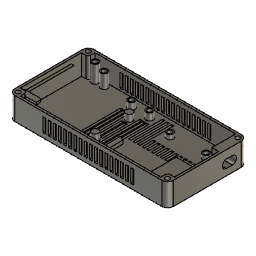
Sensors Case Bottom (Autodesk Fusion 360 design; units mm, degrees)
Autodesk Fusion 360 part; units mm, degrees
note: some values were not read from the file. Set by a fixed rule: which sketch regions a step uses.
(part 1 of 2)
sketch "Sketch1" plane through (0, 0, 0) normal (0, 0, 1) x (1, 0, 0)
  line L0 (65, 35) -> (-65, 35)
  line L1 (-70, 30) -> (-70, -30)
  line L2 (-65, -35) -> (65, -35)
  line L3 (70, -30) -> (70, 30)
  line L4 (70, 35) -> (-70, -35) construction
  line L5 (-70, 35) -> (70, -35) construction
  line L6 (-66, 44.9557) -> (-66, -54.1355) construction
  line L7 (-76.613, 31) -> (75, 31) construction
  line L8 (66, 41.9597) -> (66, -40) construction
  line L9 (75, -31) -> (-75, -31) construction
  line L10 (-62, 35) -> (-65, 35)
  line L11 (-70, 30) -> (-70, 27)
  line L12 (-70, 27) -> (-64, 27)
  line L13 (-62, 29) -> (-62, 35)
  line L14 (-62, 35) -> (-70, 27) construction
  line L15 (-70, 35) -> (-62, 27) construction
  arc A0 (-64, 27) -> (-62, 29) centre (-64, 29) ccw
  arc A1 (-65, 35) -> (-70, 30) centre (-65, 30) ccw
  arc A2 (-65, 35) -> (-70, 30) centre (-65, 30) ccw
  circle A3 centre (-66, 31) radius 3
  arc A4 (70, 30) -> (65, 35) centre (65, 30) ccw
  arc A5 (65, -35) -> (70, -30) centre (65, -30) ccw
  arc A6 (-70, -30) -> (-65, -35) centre (-65, -30) ccw
  line L16 (-64, -27) -> (-70, -27)
  line L17 (-70, -27) -> (-70, -30)
  line L18 (-65, -35) -> (-62, -35)
  line L19 (-62, -35) -> (-62, -29)
  line L20 (-62, -27) -> (-70, -35) construction
  line L21 (-70, -27) -> (-62, -35) construction
  arc A7 (-70, -30) -> (-65, -35) centre (-65, -30) ccw
  arc A8 (-62, -29) -> (-64, -27) centre (-64, -29) ccw
  circle A9 centre (-66, -31) radius 3
  line L22 (0, 0) -> (0, -13) construction
  arc A10 (64, -27) -> (62, -29) centre (64, -29) ccw
  line L23 (70, -27) -> (70, -30)
  line L24 (62, -35) -> (62, -29)
  line L25 (70, 27) -> (64, 27)
  arc A11 (70, 30) -> (65, 35) centre (65, 30) ccw
  line L26 (70, 35) -> (62, 27) construction
  arc A12 (65, -35) -> (70, -30) centre (65, -30) ccw
  line L27 (62, 35) -> (70, 27) construction
  line L28 (70, 30) -> (70, 27)
  arc A13 (65, -35) -> (70, -30) centre (65, -30) ccw
  arc A14 (62, 29) -> (64, 27) centre (64, 29) ccw
  line L29 (65, -35) -> (62, -35)
  line L30 (62, 29) -> (62, 35)
  circle A15 centre (66, -31) radius 3
  arc A16 (70, 30) -> (65, 35) centre (65, 30) ccw
  line L31 (64, -27) -> (70, -27)
  line L32 (62, -27) -> (70, -35) construction
  line L33 (70, 30) -> (70, -30)
  line L34 (62, 35) -> (65, 35)
  circle A17 centre (66, 31) radius 3
  line L35 (70, -27) -> (62, -35) construction
  line L36 (68, 33) -> (-68, 33)
  line L37 (-68, 33) -> (-68, -33)
  line L38 (-68, -33) -> (68, -33)
  line L39 (68, -33) -> (68, 33)
  line L40 (68, 33) -> (-68, -33) construction
  line L41 (-68, 33) -> (68, -33) construction
  point P0 (-66, 31)
  point P1 (-66, -31)
  point P2 (75, -31)
  point P3 (70, 35)
  point P4 (70, -35)
  point P5 (76.613, 31)
  point P6 (66, -31)
  point P7 (66, 44.9557)
  point P8 (66, 31)
  dimension "d1" = 140
  dimension "d2" = 70
  dimension "d3" = 4
  dimension "d4" = 4
  dimension "d5" = 4
  dimension "d6" = 4
  dimension "d7" = 8
  dimension "d8" = 8
  dimension "d9" = 2
  dimension "d10" = 5
  dimension "d11" = 6
  dimension "d12" = 5
  dimension "d13" = 8
  dimension "d14" = 8
  dimension "d15" = 5
  dimension "d16" = 2
  dimension "d17" = 6
  dimension "d20" = 136
  dimension "d21" = 66
  dimension "d211" = 5
  constraint horizontal L0
  constraint perpendicular L0 L1
  constraint parallel L0 L2
  constraint parallel L1 L3
  constraint coincident L4 L22.start
  constraint coincident L5 L22.start
  constraint coincident L22.start origin
  constraint vertical L6
  constraint perpendicular L3 L7
  constraint perpendicular L2 L8
  constraint perpendicular L1 L9
  constraint horizontal L10
  constraint perpendicular L10 L11
  constraint parallel L10 L12
  constraint parallel L11 L13
  constraint coincident L14 P0
  constraint coincident L15 P0
  constraint coincident L7 P0
  constraint coincident L6 P0
  constraint coincident L15.end L13
  constraint coincident L15.end L12
  constraint tangent L13 A0
  constraint tangent L12 A0
  constraint coincident L5.start L10
  constraint coincident L5.start L1
  constraint tangent L10 A1
  constraint tangent L1 A1
  constraint coincident L5.start L0
  constraint coincident L5.start L11
  constraint tangent L0 A2
  constraint tangent L11 A2
  constraint coincident P0 A3.centre
  constraint coincident P3 L0
  constraint coincident P3 L3
  constraint tangent L0 A4
  constraint tangent L3 A4
  constraint coincident L5.end L3
  constraint coincident L5.end L2
  constraint tangent L3 A5
  constraint tangent L2 A5
  constraint equal A4 A5
  constraint coincident L4.end L1
  constraint coincident L4.end L2
  constraint tangent L1 A6
  constraint tangent L2 A6
  constraint equal A4 A6
  constraint horizontal L16
  constraint perpendicular L16 L17
  constraint parallel L16 L18
  constraint parallel L17 L19
  constraint coincident L20 P1
  constraint coincident L21 P1
  constraint coincident L6 P1
  constraint coincident L9 P1
  constraint coincident L4.end L17
  constraint coincident L4.end L18
  constraint tangent L17 A7
  constraint tangent L18 A7
  constraint coincident L20.start L16
  constraint coincident L20.start L19
  constraint tangent L16 A8
  constraint tangent L19 A8
  constraint coincident P1 A9.centre
  constraint vertical L22
  constraint symmetric L5.start L22 P3
  constraint symmetric L4.end L22 P4
  constraint symmetric L6.start L22 P7
  constraint symmetric L7.start L22 P5
  constraint symmetric L9.end L22 P2
  constraint symmetric L10.start L22 L27.start
  constraint symmetric L11.end L22 L25.start
  constraint symmetric L15.end L22 L26.end
  constraint symmetric P0 L22 P8
  constraint symmetric L13.start L22 A14.start
  constraint symmetric L12.end L22 L25.end
  constraint symmetric A0 L22 A14
  constraint symmetric L0.end L22 L0.start
  constraint symmetric L1.start L22 L3.end
  constraint symmetric A1 L22 A16
  constraint symmetric A2 L22 A11
  constraint symmetric A3 L22 A17
  constraint symmetric L1.end L22 L3.start
  constraint symmetric L2.start L22 L2.end
  constraint symmetric A6 L22 A13
  constraint symmetric L20.start L22 L32.start
  constraint symmetric L16.end L22 L23.start
  constraint symmetric L18.end L22 L24.start
  constraint symmetric P1 L22 P6
  constraint symmetric A7 L22 A12
  constraint symmetric L16.start L22 A10.start
  constraint symmetric L19.end L22 A10.end
  constraint symmetric A8 L22 A10
  constraint symmetric A9 L22 A15
  constraint horizontal L36
  constraint perpendicular L36 L37
  constraint parallel L36 L38
  constraint parallel L37 L39
  constraint coincident L40 L22.start
  constraint coincident L41 L22.start
  measures "d1" distance of L4.end L5.end
  measures "d2" distance of L5.start L4.end
  measures "d3" distance of L2 L9
  measures "d4" distance of L1 L6
  measures "d5" distance of L0 L7
  measures "d6" distance of L3 L8
  measures "d7" distance of L11.end L15.end
  measures "d8" distance of L5.start L11.end
  measures "d9" radius of A0
  measures "d10" radius of A2
  measures "d11" diameter of A3
  measures "d12" radius of A4
  measures "d13" distance of L4.end L18.end
  measures "d14" distance of L16.end L4.end
  measures "d15" radius of A7
  measures "d16" radius of A8
  measures "d17" diameter of A9
  measures "d20" distance of L37.end L38.end
  measures "d21" distance of L36.end L37.end
  measures "d211" radius of A1
extrude "Extrude1" add sketch "Sketch1" along normal blind 20 contours L0 L3 A4 L25 A11 L28 L30 A16 L33 L34 A17 L36 L39 | L0 L13 L30 L36 | L0 L1 L10 L11 L12 L13 A1 A2 A3 L36 L37 | L25 A14 L30 A17 L36 L39 | L3 L25 L31 L33 L39 | L12 L13 A0 A3 L36 L37 | L2 L3 A5 L23 L24 A12 A13 L29 A15 L31 L33 L38 L39 | A10 L24 A15 L31 L38 L39 | L1 L12 L16 L37 | L1 L2 A6 L16 L17 L18 L19 A7 A9 L37 L38 | L2 L19 L24 L38 | L16 L19 A8 A9 L37 L38 makes body 1
sketch "Sketch3" plane through (0, 0, 0) normal (0, 0, -1) x (1, 0, 0)
  circle A0 centre (-66, -31) radius 3
  circle A1 centre (66, 31) radius 3
  line L0 (-62, 33) -> (62, 33)
  line L1 (62, 33) -> (62, 29)
  arc A2 (62, 29) -> (64, 27) centre (64, 29) ccw
  line L2 (64, 27) -> (68, 27)
  line L3 (68, 27) -> (68, -27)
  line L4 (68, -27) -> (64, -27)
  arc A3 (64, -27) -> (62, -29) centre (64, -29) ccw
  line L5 (62, -29) -> (62, -33)
  line L6 (62, -33) -> (-62, -33)
  line L7 (-62, -33) -> (-62, -29)
  arc A4 (-62, -29) -> (-64, -27) centre (-64, -29) ccw
  line L8 (-64, -27) -> (-68, -27)
  line L9 (-68, -27) -> (-68, 27)
  line L10 (-68, 27) -> (-64, 27)
  arc A5 (-64, 27) -> (-62, 29) centre (-64, 29) ccw
  line L11 (-62, 29) -> (-62, 33)
  circle A6 centre (66, -31) radius 3
  circle A7 centre (-66, 31) radius 3
  line L12 (-65, -35) -> (65, -35)
  arc A8 (65, -35) -> (70, -30) centre (65, -30) ccw
  line L13 (70, -30) -> (70, 30)
  arc A9 (70, 30) -> (65, 35) centre (65, 30) ccw
  line L14 (65, 35) -> (-65, 35)
  arc A10 (-65, 35) -> (-70, 30) centre (-65, 30) ccw
  line L15 (-70, 30) -> (-70, -30)
  arc A11 (-70, -30) -> (-65, -35) centre (-65, -30) ccw
  line L16 (-68, -35) -> (68, -35)
  line L17 (70, -33) -> (70, 33)
  line L18 (68, 35) -> (-68, 35)
  line L19 (-70, 33) -> (-70, -33)
  line L20 (-70, -35) -> (70, 35) construction
  line L21 (70, -35) -> (-70, 35) construction
  arc A12 (-70, -33) -> (-68, -35) centre (-68, -33) ccw
  arc A13 (-68, 35) -> (-70, 33) centre (-68, 33) ccw
  arc A14 (70, 33) -> (68, 35) centre (68, 33) ccw
  arc A15 (68, -35) -> (70, -33) centre (68, -33) ccw
  dimension "d22" = 140
  dimension "d23" = 70
  dimension "d24" = 2
  constraint horizontal L16
  constraint perpendicular L16 L17
  constraint parallel L16 L18
  constraint parallel L17 L19
  constraint coincident L20 origin
  constraint coincident L21 origin
  constraint coincident L20.start L16
  constraint coincident L20.start L19
  constraint tangent L16 A12
  constraint tangent L19 A12
  constraint coincident L21.end L19
  constraint coincident L21.end L18
  constraint tangent L19 A13
  constraint tangent L18 A13
  constraint equal A12 A13
  constraint coincident L20.end L18
  constraint coincident L20.end L17
  constraint tangent L18 A14
  constraint tangent L17 A14
  constraint equal A12 A14
  constraint coincident L21.start L17
  constraint coincident L21.start L16
  constraint tangent L17 A15
  constraint tangent L16 A15
  constraint equal A12 A15
  measures "d22" distance of L20.end L21.end
  measures "d23" distance of L21.start L20.end
  measures "d24" radius of A12
extrude "Extrude2" add sketch "Sketch3" against normal blind 2 contours L0 L1 A2 L2 L3 L4 A3 L5 L6 L7 A4 L8 L9 L10 A5 L11 | L12 A8 L13 A9 L14 A10 L15 A11 L16 L17 L18 L19 bodies 1
sketch "Sketch22" plane through (0, 0, 2) normal (0, 0, 1) x (-1, 0, 0)
  line L0 (-62, 33) -> (-62, 29)
  arc A0 (-64, 27) -> (-62, 29) centre (-64, 29) ccw
  line L1 (-64, 27) -> (-68, 27)
  line L2 (-68, 27) -> (-68, -27)
  line L3 (-68, -27) -> (-64, -27)
  arc A1 (-62, -29) -> (-64, -27) centre (-64, -29) ccw
  line L4 (-62, -29) -> (-62, -33)
  line L5 (-62, -33) -> (62, -33)
  line L6 (62, -33) -> (62, -29)
  arc A2 (64, -27) -> (62, -29) centre (64, -29) ccw
  line L7 (64, -27) -> (68, -27)
  line L8 (68, -27) -> (68, 27)
  line L9 (68, 27) -> (64, 27)
  arc A3 (62, 29) -> (64, 27) centre (64, 29) ccw
  line L10 (62, 29) -> (62, 33)
  line L11 (62, 33) -> (-62, 33)
  line L12 (-62, 27) -> (-62, 2)
  line L13 (-62, 2) -> (-68, 2)
  line L14 (-68, 2) -> (-68, 27)
  line L15 (-64.3335, 27) -> (-64.3335, 27.5858)
  line L16 (-64.3335, 27.5858) -> (-62.5858, 27.5858)
  line L17 (-62, 27.5858) -> (-62, 27)
  line L18 (-62.5858, 27.5858) -> (-62.5858, 29.0477)
  line L19 (-62.5858, 29.0477) -> (-62, 29.0477)
  line L20 (-62, 29.0477) -> (-62, 27)
  line L21 (-68, 27) -> (-64.3335, 27)
  constraint horizontal L21
  constraint vertical L12
  constraint horizontal L13
  constraint vertical L14
  constraint coincident L1.end L2.start
  constraint vertical L15
  constraint horizontal L16
  constraint vertical L17
  constraint vertical L18
  constraint horizontal L19
  constraint vertical L20
  constraint coincident A0 L16.end
extrude "Extrude21" add sketch "Sketch22" along normal blind 5 contours A0 L1 L2 L12 L13 L14 L17 L20 L21 bodies 1
sketch "Sketch4" plane through (0, 0, 2) normal (0, 0, 1) x (-1, 0, 0)
  line L0 (-62, 33) -> (-62, 2)
  line L1 (-68, 2) -> (-68, -27)
  line L2 (-68, -27) -> (-64, -27)
  arc A0 (-62, -29) -> (-64, -27) centre (-64, -29) ccw
  line L3 (-62, -29) -> (-62, -33)
  line L4 (-62, -33) -> (62, -33)
  line L5 (62, -33) -> (62, -29)
  arc A1 (64, -27) -> (62, -29) centre (64, -29) ccw
  line L6 (64, -27) -> (68, -27)
  line L7 (68, -27) -> (68, 27)
  line L8 (68, 27) -> (64, 27)
  arc A2 (62, 29) -> (64, 27) centre (64, 29) ccw
  line L9 (62, 29) -> (62, 33)
  line L10 (62, 33) -> (-62, 33)
  line L11 (-45, 1.5) -> (-68, 1.5)
  line L12 (-68, 1.5) -> (-68, 0.5)
  line L13 (-68, 0.5) -> (-45, 0.5)
  line L14 (-45, 0.5) -> (-45, 1.5)
  line L15 (-62, 2) -> (-68, 2)
  dimension "d119" = 1
  dimension "d202" = 31.5
  constraint horizontal L11
  constraint vertical L12
  constraint horizontal L13
  constraint vertical L14
  measures "d119" distance of L11.end L12.end
  measures "d202" distance of L10 L11
extrude "Extrude3" add sketch "Sketch4" along normal blind 8.5 contours L1 L11 L12 L13 L14 bodies 1
sketch "Sketch5" plane through (0, 0, 10.5) normal (0, 0, 1) x (-1, 0, 0)
  line L0 (-45, 0.5) -> (-45, 1.5)
  line L1 (-45, 1.5) -> (-68, 1.5)
  line L2 (-68, 1.5) -> (-68, 0.5)
  line L3 (-68, 0.5) -> (-45, 0.5)
  line L4 (-45, 0.5) -> (-68, 0.5)
  line L5 (-68, 0.5) -> (-68, 27)
  line L6 (-68, 27) -> (-64, 27)
  line L7 (-45, 27) -> (-45, 0.5)
  line L8 (-62, 29) -> (-62, 33)
  line L9 (-62, 33) -> (-45, 33)
  line L10 (-45, 33) -> (-45, 27)
  arc A0 (-64, 27) -> (-62, 29) centre (-64, 29) ccw
  point P0 (-68, 27)
  point P1 (-62, 33)
  dimension "d29" = 2
  constraint horizontal L4
  constraint vertical L5
  constraint horizontal L6
  constraint vertical L7
  constraint coincident L0.start L3.end
  constraint vertical L8
  constraint horizontal L9
  constraint vertical L10
  constraint coincident L7.start L6
  constraint tangent L8 A0
  constraint tangent L6 A0
  constraint coincident P0 L5.end
  constraint coincident P1 L8.end
  measures "d29" radius of A0
extrude "Extrude4" add sketch "Sketch5" along normal blind 1 bodies 1
fillet "Fillet1" radius 2 1 edges at (56.5, -0.5, 11.5) on bodies 1
sketch "Sketch26" plane through (0, -35, 0) normal (0, -1, 0) x (1, 0, 0)
  line L0 (65, 0) -> (65, 20)
  line L1 (65, 20) -> (-65, 20)
  line L2 (-65, 20) -> (-65, 0)
  line L3 (-65, 0) -> (65, 0)
  line L4 (0, 0) -> (0, 20) construction
  line L5 (42, 16) -> (-42, 16)
  line L6 (-42, 16) -> (-42, 4)
  line L7 (-42, 4) -> (42, 4)
  line L8 (42, 4) -> (42, 16)
  line L9 (42, 16) -> (-42, 4) construction
  line L10 (-42, 16) -> (42, 4) construction
  line L11 (-40, 16) -> (-40, 4)
  line L12 (-35.4444, 16) -> (-35.4444, 4)
  line L13 (-37.4444, 16) -> (-37.4444, 4)
  line L14 (-30.8889, 16) -> (-30.8889, 4)
  line L15 (-32.8889, 16) -> (-32.8889, 4)
  line L16 (-26.3333, 16) -> (-26.3333, 4)
  line L17 (-28.3333, 16) -> (-28.3333, 4)
  line L18 (-21.7778, 16) -> (-21.7778, 4)
  line L19 (-23.7778, 16) -> (-23.7778, 4)
  line L20 (-17.2222, 16) -> (-17.2222, 4)
  line L21 (-19.2222, 16) -> (-19.2222, 4)
  line L22 (-12.6667, 16) -> (-12.6667, 4)
  line L23 (-14.6667, 16) -> (-14.6667, 4)
  line L24 (-8.1111, 16) -> (-8.1111, 4)
  line L25 (-10.1111, 16) -> (-10.1111, 4)
  line L26 (-3.5556, 16) -> (-3.5556, 4)
  line L27 (-5.5556, 16) -> (-5.5556, 4)
  line L28 (1, 16) -> (1, 4)
  line L29 (-1, 16) -> (-1, 4)
  line L30 (5.5556, 16) -> (5.5556, 4)
  line L31 (3.5556, 16) -> (3.5556, 4)
  line L32 (10.1111, 16) -> (10.1111, 4)
  line L33 (8.1111, 16) -> (8.1111, 4)
  line L34 (14.6667, 16) -> (14.6667, 4)
  line L35 (12.6667, 16) -> (12.6667, 4)
  line L36 (19.2222, 16) -> (19.2222, 4)
  line L37 (17.2222, 16) -> (17.2222, 4)
  line L38 (23.7778, 16) -> (23.7778, 4)
  line L39 (21.7778, 16) -> (21.7778, 4)
  line L40 (28.3333, 16) -> (28.3333, 4)
  line L41 (26.3333, 16) -> (26.3333, 4)
  line L42 (32.8889, 16) -> (32.8889, 4)
  line L43 (30.8889, 16) -> (30.8889, 4)
  line L44 (37.4444, 16) -> (37.4444, 4)
  line L45 (35.4444, 16) -> (35.4444, 4)
  line L46 (42, 16) -> (42, 4)
  line L47 (40, 16) -> (40, 4)
  point P0 (0, 10)
  dimension "d222" = 84
  dimension "d223" = 12
  dimension "d224" = 2
  dimension "d227" = 82
  dimension "d228" = 0
  constraint coincident L4.start origin
  constraint midpoint L1 L4.end
  constraint horizontal L5
  constraint perpendicular L5 L6
  constraint parallel L5 L7
  constraint parallel L6 L8
  constraint coincident L9 P0
  constraint coincident L10 P0
  constraint midpoint L4 P0
  constraint coincident L5 L11.start
  constraint coincident L7 L11.end
  constraint perpendicular L7 L11
  measures "d222" distance of L6.end L7.end
  measures "d223" distance of L5.end L6.end
  measures "d224" distance of L6 L11
extrude "Extrude25" cut sketch "Sketch26" against normal blind 70 contours L5 L7 L44 L47 | L5 L7 L42 L45 | L5 L7 L40 L43 | L5 L7 L38 L41 | L5 L7 L36 L39 | L5 L7 L34 L37 | L5 L7 L32 L35 | L5 L7 L30 L33 | L5 L7 L28 L31 | L5 L7 L26 L29 | L5 L7 L24 L27 | L5 L7 L22 L25 | L5 L7 L20 L23 | L5 L7 L18 L21 | L5 L7 L16 L19 | L5 L7 L14 L17 | L5 L7 L12 L15 | L5 L7 L11 L13 bodies 1
sketch "Sketch9" plane through (0, 0, 2) normal (0, 0, 1) x (-1, 0, 0)
  line L0 (-68, 1.5) -> (-45, 1.5)
  line L1 (-45, 1.5) -> (-45, 0.5)
  line L2 (-45, 0.5) -> (-68, 0.5)
  line L3 (-68, 0.5) -> (-68, -27)
  line L4 (-68, -27) -> (-64, -27)
  arc A0 (-62, -29) -> (-64, -27) centre (-64, -29) ccw
  line L5 (-62, -29) -> (-62, -33)
  line L6 (-62, -33) -> (62, -33)
  line L7 (62, -33) -> (62, -29)
  arc A1 (64, -27) -> (62, -29) centre (64, -29) ccw
  line L8 (64, -27) -> (68, -27)
  line L9 (68, -27) -> (68, 27)
  line L10 (68, 27) -> (64, 27)
  arc A2 (62, 29) -> (64, 27) centre (64, 29) ccw
  line L11 (62, 29) -> (62, 33)
  line L12 (62, 33) -> (-62, 33)
  line L13 (-62, 33) -> (-62, 2)
  line L14 (-68, 2) -> (-68, 1.5)
  circle A3 centre (50, -29) radius 2
  circle A4 centre (50, -29) radius 3
  line L15 (-62, 2) -> (-68, 2)
  dimension "d86" = 4
  dimension "d87" = 6
  dimension "d142" = 4
  dimension "d143" = 12
  constraint concentric A3 A4
  measures "d86" diameter of A3
  measures "d87" diameter of A4
  measures "d142" distance of L6 A3.centre
  measures "d143" distance of L7 A3.centre
extrude "Extrude9" add sketch "Sketch9" along normal blind 12 separate body contours A4 makes body 2
sketch "Sketch10" plane through (-68, 0, 0) normal (1, 0, 0) x (0, 1, 0)
  line L0 (-27, 2) -> (27, 2)
  line L1 (27, 2) -> (27, 20)
  line L2 (27, 20) -> (-27, 20)
  line L3 (-27, 20) -> (-27, 2)
  line L4 (-25, 14) -> (18, 14)
  line L5 (18, 14) -> (18, 16)
  line L6 (18, 16) -> (-25, 16)
  line L7 (-25, 16) -> (-25, 14)
  dimension "d90" = 2
  dimension "d91" = 43
  dimension "d92" = 2
  dimension "d96" = 4
  constraint horizontal L4
  constraint vertical L5
  constraint horizontal L6
  constraint vertical L7
  measures "d90" distance of L3 L6.end
  measures "d91" distance of L5.end L6.end
  measures "d92" distance of L4.start L6.end
  measures "d96" distance of L2 L6
extrude "Extrude10" add sketch "Sketch10" along normal blind 2.5 contours L4 L5 L6 L7 bodies 1
chamfer "Chamfer1" distance 2 angle 45 1 edges at (-65.5, -3.5, 14) on bodies 1
sketch "Sketch11" plane through (0, 0, 2) normal (0, 0, 1) x (-1, 0, 0)
  line L0 (-68, 1.5) -> (-45, 1.5)
  line L1 (-45, 1.5) -> (-45, 0.5)
  line L2 (-45, 0.5) -> (-68, 0.5)
  line L3 (-68, 0.5) -> (-68, -27)
  line L4 (-68, -27) -> (-64, -27)
  arc A0 (-62, -29) -> (-64, -27) centre (-64, -29) ccw
  line L5 (-62, -29) -> (-62, -33)
  line L6 (-62, -33) -> (62, -33)
  line L7 (62, -33) -> (62, -29)
  arc A1 (64, -27) -> (62, -29) centre (64, -29) ccw
  line L8 (64, -27) -> (68, -27)
  line L9 (68, -27) -> (68, 27)
  line L10 (68, 27) -> (64, 27)
  arc A2 (62, 29) -> (64, 27) centre (64, 29) ccw
  line L11 (62, 29) -> (62, 33)
  line L12 (62, 33) -> (-62, 33)
  line L13 (-62, 33) -> (-62, 2)
  line L14 (-68, 2) -> (-68, 1.5)
  circle A3 centre (21.9294, -25) radius 2
  circle A4 centre (5.9294, -25) radius 2
  circle A5 centre (5.9294, -25) radius 3
  circle A6 centre (21.9294, -25) radius 3
  circle A7 centre (5.9294, 25) radius 2
  circle A8 centre (5.9294, 25) radius 3
  circle A9 centre (21.9294, 25) radius 2
  circle A10 centre (21.9294, 25) radius 3
  line L15 (5.9294, 25) -> (5.9294, -25) construction
  line L16 (21.9294, -25) -> (21.9294, 25) construction
  line L17 (0, 0) -> (27, 0) construction
  line L18 (-62, 2) -> (-68, 2)
  point P0 (21.9294, 0)
  point P1 (5.9294, 0)
  dimension "d97" = 4
  dimension "d98" = 4
  dimension "d99" = 6
  dimension "d100" = 6
  dimension "d101" = 4
  dimension "d102" = 6
  dimension "d103" = 4
  dimension "d104" = 6
  dimension "d151" = 16
  dimension "d154" = 25
  dimension "d155" = 25
  constraint concentric A4 A5
  constraint concentric A3 A6
  constraint concentric A7 A8
  constraint concentric A9 A10
  constraint coincident A7.centre A8.centre
  constraint coincident A4.centre A5.centre
  constraint vertical L15
  constraint coincident A3.centre A6.centre
  constraint coincident A9.centre A10.centre
  constraint vertical L16
  constraint coincident L17.start origin
  constraint horizontal L17
  constraint midpoint L16 P0
  constraint midpoint L15 P1
  constraint coincident L17 P0
  constraint coincident L17 P1
  measures "d97" diameter of A3
  measures "d98" diameter of A4
  measures "d99" diameter of A5
  measures "d100" diameter of A6
  measures "d101" diameter of A7
  measures "d102" diameter of A8
  measures "d103" diameter of A9
  measures "d104" diameter of A10
  measures "d151" distance of L15 L16
  measures "d154" distance of A4.centre P1
  measures "d155" distance of A3.centre L17
extrude "Extrude11" add sketch "Sketch11" along normal blind 6 contours A5 | A6 | A8 | A10 bodies 1
sketch "Sketch12" plane through (0, 0, 2) normal (0, 0, 1) x (-1, 0, 0)
  circle A0 centre (21.9294, -25) radius 3
  circle A1 centre (5.9294, -25) radius 3
  line L0 (-68, 1.5) -> (-45, 1.5)
  line L1 (-45, 1.5) -> (-45, 0.5)
  line L2 (-45, 0.5) -> (-68, 0.5)
  line L3 (-68, 0.5) -> (-68, -27)
  line L4 (-68, -27) -> (-64, -27)
  arc A2 (-62, -29) -> (-64, -27) centre (-64, -29) ccw
  line L5 (-62, -29) -> (-62, -33)
  line L6 (-62, -33) -> (62, -33)
  line L7 (62, -33) -> (62, -29)
  arc A3 (64, -27) -> (62, -29) centre (64, -29) ccw
  line L8 (64, -27) -> (68, -27)
  line L9 (68, -27) -> (68, 27)
  line L10 (68, 27) -> (64, 27)
  arc A4 (62, 29) -> (64, 27) centre (64, 29) ccw
  line L11 (62, 29) -> (62, 33)
  line L12 (62, 33) -> (-62, 33)
  line L13 (-62, 33) -> (-62, 2)
  line L14 (-68, 2) -> (-68, 1.5)
  circle A5 centre (5.9294, 25) radius 3
  circle A6 centre (21.9294, 25) radius 3
  circle A7 centre (13.9294, -15) radius 3
  circle A8 centre (13.9294, 15) radius 3
  line L15 (5.9294, 25) -> (21.9294, 25) construction
  line L16 (13.9294, 25) -> (13.9294, 15) construction
  line L17 (5.9294, -25) -> (21.9294, -25) construction
  line L18 (21.9294, -25) -> (13.9294, -25)
  line L19 (13.9294, -15) -> (13.9294, -25) construction
  line L20 (-62, 2) -> (-68, 2)
  dimension "d115" = 6
  dimension "d116" = 6
  dimension "d153" = 10
  dimension "d156" = 10
  constraint coincident A5.centre L15.start
  constraint coincident A6.centre L15.end
  constraint midpoint L15 L16.start
  constraint coincident A8.centre L16.end
  constraint perpendicular L15 L16
  constraint coincident A1.centre L17.start
  constraint coincident A0.centre L17.end
  constraint midpoint L17 L18.end
  constraint coincident A7.centre L19.start
  constraint perpendicular L17 L19
  measures "d115" diameter of A7
  measures "d116" diameter of A8
  measures "d153" distance of A7.centre L17
  measures "d156" distance of A8.centre L15
extrude "Extrude12" add sketch "Sketch12" along normal blind 6 contours A7 | A8 bodies 1
sketch "Sketch13" plane through (0, 0, 20) normal (0, 0, 1) x (-1, 0, 0)
  line L0 (-62, 33) -> (62, 33)
  line L1 (62, 33) -> (62, 29)
  arc A0 (62, 29) -> (64, 27) centre (64, 29) ccw
  line L2 (64, 27) -> (68, 27)
  line L3 (68, 27) -> (68, -27)
  line L4 (68, -27) -> (64, -27)
  arc A1 (64, -27) -> (62, -29) centre (64, -29) ccw
  line L5 (62, -29) -> (62, -33)
  line L6 (62, -33) -> (-62, -33)
  line L7 (-62, -33) -> (-62, -29)
  arc A2 (-62, -29) -> (-64, -27) centre (-64, -29) ccw
  line L8 (-64, -27) -> (-68, -27)
  line L9 (-68, -27) -> (-68, 27)
  line L10 (-68, 27) -> (-64, 27)
  arc A3 (-64, 27) -> (-62, 29) centre (-64, 29) ccw
  line L11 (-62, 29) -> (-62, 33)
  circle A4 centre (-66, -31) radius 3
  circle A5 centre (66, -31) radius 3
  circle A6 centre (-66, 31) radius 3
  circle A7 centre (66, 31) radius 3
  line L12 (-65, -35) -> (65, -35)
  arc A8 (65, -35) -> (70, -30) centre (65, -30) ccw
  line L13 (70, -30) -> (70, 30)
  arc A9 (70, 30) -> (65, 35) centre (65, 30) ccw
  line L14 (65, 35) -> (-65, 35)
  arc A10 (-65, 35) -> (-70, 30) centre (-65, 30) ccw
  line L15 (-70, 30) -> (-70, -30)
  arc A11 (-70, -30) -> (-65, -35) centre (-65, -30) ccw
  circle A12 centre (66, -31) radius 2
  circle A13 centre (66, 31) radius 2
  circle A14 centre (-66, 31) radius 2
  circle A15 centre (-66, -31) radius 2
  dimension "d121" = 4
  dimension "d122" = 4
  dimension "d123" = 4
  dimension "d124" = 4
  constraint concentric A5 A12
  constraint concentric A7 A13
  constraint concentric A6 A14
  constraint concentric A4 A15
  measures "d121" diameter of A12
  measures "d122" diameter of A13
  measures "d123" diameter of A14
  measures "d124" diameter of A15
extrude "Extrude13" add sketch "Sketch13" against normal blind 6 contours A4 | A5 | A6 | A7 bodies 1
chamfer "Chamfer2" distance 1 angle 45 4 edges at (-64.1353, -30.2768, 14) (-64.1353, 31.7232, 14) (67.8647, -30.2768, 14) (67.8647, 31.7232, 14) on bodies 1
sketch "Sketch16" plane through (0, 0, 2) normal (0, 0, 1) x (-1, 0, 0)
  circle A0 centre (13.9294, -15) radius 3
  circle A1 centre (21.9294, -25) radius 3
  circle A2 centre (5.9294, -25) radius 3
  line L0 (-68, 1.5) -> (-45, 1.5)
  line L1 (-45, 1.5) -> (-45, 0.5)
  line L2 (-45, 0.5) -> (-68, 0.5)
  line L3 (-68, 0.5) -> (-68, -27)
  line L4 (-68, -27) -> (-64, -27)
  arc A3 (-62, -29) -> (-64, -27) centre (-64, -29) ccw
  line L5 (-62, -29) -> (-62, -33)
  line L6 (-62, -33) -> (62, -33)
  line L7 (62, -33) -> (62, -29)
  arc A4 (64, -27) -> (62, -29) centre (64, -29) ccw
  line L8 (64, -27) -> (68, -27)
  line L9 (68, -27) -> (68, 27)
  line L10 (68, 27) -> (64, 27)
  arc A5 (62, 29) -> (64, 27) centre (64, 29) ccw
  line L11 (62, 29) -> (62, 33)
  line L12 (62, 33) -> (-62, 33)
  line L13 (-62, 33) -> (-62, 2)
  line L14 (-68, 2) -> (-68, 1.5)
  circle A6 centre (5.9294, 25) radius 3
  circle A7 centre (21.9294, 25) radius 3
  line L15 (33.1094, 24.8906) -> (29.1094, 24.8906)
  line L16 (29.1094, 24.8906) -> (29.1094, 28.8906)
  line L17 (29.1094, 28.8906) -> (33.1094, 28.8906)
  line L18 (33.1094, 28.8906) -> (33.1094, 24.8906)
  line L19 (33.1094, 24.8906) -> (29.1094, 28.8906) construction
  line L20 (29.1094, 24.8906) -> (33.1094, 28.8906) construction
  line L21 (33.1094, 26.8906) -> (32.1094, 26.8906)
  line L22 (31.1094, 25.8906) -> (31.1094, 24.8906)
  arc A8 (32.1094, 26.8906) -> (31.1094, 25.8906) centre (32.1094, 25.8906) ccw
  circle A9 centre (13.9294, 15) radius 3
  line L23 (-62, 2) -> (-68, 2)
  point P0 (31.1094, 26.8906)
  dimension "d134" = 1
  constraint horizontal L15
  constraint perpendicular L15 L16
  constraint parallel L15 L17
  constraint parallel L16 L18
  constraint coincident L19 P0
  constraint coincident L20 P0
  constraint midpoint L18 L21.start
  constraint midpoint L15 L22.end
  constraint tangent L22 A8
  constraint tangent L21 A8
  measures "d134" radius of A8
extrude "Extrude15" add sketch "Sketch16" along normal blind 2 contours L15 L16 L17 L18 L21 L22 A8 bodies 1
chamfer "Chamfer3" distance 2 angle 45 4 edges at (-29.1094, -26.8906, 2) (-30.1094, -24.8906, 2) (-31.1094, -28.8906, 2) (-33.1094, -27.8906, 2) on bodies 1
sketch "Sketch17" plane through (0, 0, 2) normal (0, 0, 1) x (-1, 0, 0)
  circle A0 centre (21.9294, 25) radius 3
  circle A1 centre (5.9294, 25) radius 3
  line L0 (-68, 1.5) -> (-45, 1.5)
  line L1 (-45, 1.5) -> (-45, 0.5)
  line L2 (-45, 0.5) -> (-68, 0.5)
  line L3 (-68, 0.5) -> (-68, -27)
  line L4 (-68, -27) -> (-64, -27)
  arc A2 (-62, -29) -> (-64, -27) centre (-64, -29) ccw
  line L5 (-62, -29) -> (-62, -33)
  line L6 (-62, -33) -> (62, -33)
  line L7 (62, -33) -> (62, -29)
  arc A3 (64, -27) -> (62, -29) centre (64, -29) ccw
  line L8 (64, -27) -> (68, -27)
  line L9 (68, -27) -> (68, 27)
  line L10 (68, 27) -> (64, 27)
  arc A4 (62, 29) -> (64, 27) centre (64, 29) ccw
  line L11 (62, 29) -> (62, 33)
  line L12 (62, 33) -> (-62, 33)
  line L13 (-62, 33) -> (-62, 2)
  line L14 (-68, 2) -> (-68, 1.5)
  circle A5 centre (5.9294, -25) radius 3
  circle A6 centre (21.9294, -25) radius 3
  circle A7 centre (13.9294, -15) radius 3
  line L15 (31.1094, 25.8906) -> (31.1094, 22.8906)
  line L16 (31.1094, 22.8906) -> (27.1094, 22.8906)
  line L17 (27.1094, 22.8906) -> (27.1094, 30.8906)
  line L18 (27.1094, 30.8906) -> (35.1094, 30.8906)
  line L19 (35.1094, 30.8906) -> (35.1094, 26.8906)
  line L20 (35.1094, 26.8906) -> (32.1094, 26.8906)
  arc A8 (32.1094, 26.8906) -> (31.1094, 25.8906) centre (32.1094, 25.8906) ccw
  line L21 (64, 28) -> (53, 28)
  line L22 (53, 28) -> (53, 27)
  line L23 (53, 27) -> (64, 27)
  line L24 (64, 27) -> (64, 28)
  circle A9 centre (13.9294, 15) radius 3
  line L25 (-62, 2) -> (-68, 2)
  constraint horizontal L21
  constraint vertical L22
  constraint horizontal L23
  constraint vertical L24
extrude "Extrude16" add sketch "Sketch17" along normal blind 13 contours A4 L21 L22 L23 bodies 1
sketch "Sketch18" plane through (0, 0, 15) normal (0, 0, 1) x (-1, 0, 0)
  line L0 (62.2679, 28) -> (53, 28)
  line L1 (53, 28) -> (53, 27)
  line L2 (53, 27) -> (64, 27)
  arc A0 (62.2679, 28) -> (64, 27) centre (64, 29) ccw
  line L3 (53, 28) -> (68, 28)
  line L4 (68, 28) -> (68, 23)
  line L5 (68, 23) -> (53, 23)
  line L6 (53, 23) -> (53, 28)
  dimension "d146" = 15
  dimension "d147" = 5
  constraint horizontal L3
  constraint vertical L4
  constraint horizontal L5
  constraint vertical L6
  constraint coincident L0.end L1.start
  measures "d146" distance of L0.end L3.end
  measures "d147" distance of L0.end L5.end
extrude "Extrude17" add sketch "Sketch18" along normal blind 2 bodies 1
chamfer "Chamfer4" distance 2 angle 45 1 edges at (-59.75, -23, 15) on bodies 1
sketch "Sketch19" plane through (0, 0, 2) normal (0, 0, 1) x (-1, 0, 0)
  line L0 (31.1094, 25.8906) -> (31.1094, 22.8906)
  line L1 (31.1094, 22.8906) -> (27.1094, 22.8906)
  line L2 (27.1094, 22.8906) -> (27.1094, 30.8906)
  line L3 (27.1094, 30.8906) -> (35.1094, 30.8906)
  line L4 (35.1094, 30.8906) -> (35.1094, 26.8906)
  line L5 (35.1094, 26.8906) -> (32.1094, 26.8906)
  arc A0 (32.1094, 26.8906) -> (31.1094, 25.8906) centre (32.1094, 25.8906) ccw
  circle A1 centre (13.9294, 15) radius 3
  circle A2 centre (13.9294, -15) radius 3
  circle A3 centre (21.9294, -25) radius 3
  circle A4 centre (5.9294, -25) radius 3
  line L6 (68, 27) -> (53, 27)
  line L7 (53, 27) -> (53, 28)
  line L8 (53, 28) -> (62.2679, 28)
  arc A5 (62, 29) -> (62.2679, 28) centre (64, 29) ccw
  line L9 (62, 29) -> (62, 33)
  line L10 (62, 33) -> (-62, 33)
  line L11 (-62, 33) -> (-62, 2)
  line L12 (-68, 2) -> (-68, 1.5)
  line L13 (-68, 1.5) -> (-45, 1.5)
  line L14 (-45, 1.5) -> (-45, 0.5)
  line L15 (-45, 0.5) -> (-68, 0.5)
  line L16 (-68, 0.5) -> (-68, -27)
  line L17 (-68, -27) -> (-64, -27)
  arc A6 (-62, -29) -> (-64, -27) centre (-64, -29) ccw
  line L18 (-62, -29) -> (-62, -33)
  line L19 (-62, -33) -> (62, -33)
  line L20 (62, -33) -> (62, -29)
  arc A7 (64, -27) -> (62, -29) centre (64, -29) ccw
  line L21 (64, -27) -> (68, -27)
  line L22 (68, -27) -> (68, 27)
  circle A8 centre (5.9294, 25) radius 3
  circle A9 centre (21.9294, 25) radius 3
  circle A10 centre (-49.5, -19.5) radius 2
  circle A11 centre (-49.5, -19.5) radius 3
  circle A12 centre (-17.5, -19.5) radius 2
  circle A13 centre (-17.5, -19.5) radius 3
  line L23 (-62, 2) -> (-68, 2)
  dimension "d165" = 4
  dimension "d166" = 6
  dimension "d167" = 4
  dimension "d168" = 6
  dimension "d169" = 32
  dimension "d170" = 13.5
  dimension "d171" = 12.5
  dimension "d172" = 13.5
  constraint concentric A10 A11
  constraint concentric A12 A13
  measures "d165" diameter of A10
  measures "d166" diameter of A11
  measures "d167" diameter of A12
  measures "d168" diameter of A13
  measures "d169" distance of A10.centre A12.centre
  measures "d170" distance of L19 A10.centre
  measures "d171" distance of L18 A10.centre
  measures "d172" distance of L19 A12.centre
extrude "Extrude18" add sketch "Sketch19" along normal blind 4 contours A11 | A13 bodies 1
sketch "Sketch20" plane through (0, 0, 2) normal (0, 0, 1) x (-1, 0, 0)
  circle A0 centre (-17.5, -19.5) radius 3
  line L0 (31.1094, 25.8906) -> (31.1094, 22.8906)
  line L1 (31.1094, 22.8906) -> (27.1094, 22.8906)
  line L2 (27.1094, 22.8906) -> (27.1094, 30.8906)
  line L3 (27.1094, 30.8906) -> (35.1094, 30.8906)
  line L4 (35.1094, 30.8906) -> (35.1094, 26.8906)
  line L5 (35.1094, 26.8906) -> (32.1094, 26.8906)
  arc A1 (32.1094, 26.8906) -> (31.1094, 25.8906) centre (32.1094, 25.8906) ccw
  circle A2 centre (13.9294, 15) radius 3
  circle A3 centre (13.9294, -15) radius 3
  circle A4 centre (21.9294, -25) radius 3
  circle A5 centre (5.9294, -25) radius 3
  line L6 (68, 27) -> (53, 27)
  line L7 (53, 27) -> (53, 28)
  line L8 (53, 28) -> (62.2679, 28)
  arc A6 (62, 29) -> (62.2679, 28) centre (64, 29) ccw
  line L9 (62, 29) -> (62, 33)
  line L10 (62, 33) -> (-62, 33)
  line L11 (-62, 33) -> (-62, 2)
  line L12 (-68, 2) -> (-68, 1.5)
  line L13 (-68, 1.5) -> (-45, 1.5)
  line L14 (-45, 1.5) -> (-45, 0.5)
  line L15 (-45, 0.5) -> (-68, 0.5)
  line L16 (-68, 0.5) -> (-68, -27)
  line L17 (-68, -27) -> (-64, -27)
  arc A7 (-62, -29) -> (-64, -27) centre (-64, -29) ccw
  line L18 (-62, -29) -> (-62, -33)
  line L19 (-62, -33) -> (62, -33)
  line L20 (62, -33) -> (62, -29)
  arc A8 (64, -27) -> (62, -29) centre (64, -29) ccw
  line L21 (64, -27) -> (68, -27)
  line L22 (68, -27) -> (68, 27)
  circle A9 centre (5.9294, 25) radius 3
  circle A10 centre (21.9294, 25) radius 3
  circle A11 centre (-49.5, -19.5) radius 3
  line L23 (-68, -27) -> (-64, -27)
  line L24 (-64, -27) -> (-64, -12)
  line L25 (-64, -12) -> (-68, -12)
  line L26 (-68, -12) -> (-68, -27)
  line L27 (-64, -12) -> (-62, -12)
  line L28 (-62, -12) -> (-62, -14.5)
  line L29 (-62, -14.5) -> (-64, -14.5)
  line L30 (-64, -14.5) -> (-64, -12)
  line L31 (-62, -24.55) -> (-64, -24.55)
  line L32 (-62, -24.55) -> (-64, -24.55)
  line L33 (-64, -24.55) -> (-64, -29.55)
  line L34 (-64, -29.55) -> (-62, -29.55)
  line L35 (-62, -29.55) -> (-62, -24.55)
  line L36 (-62, -24.55) -> (-64, -24.55)
  line L37 (-64, -24.55) -> (-64, -14.5)
  line L38 (-64, -14.5) -> (-62, -14.5)
  line L39 (-62, -14.5) -> (-62, -24.55)
  line L40 (-62, 2) -> (-68, 2)
  dimension "d181" = 4
  dimension "d182" = 15
  dimension "d185" = 2
  dimension "d186" = 2.5
  dimension "d188" = 2
  dimension "d189" = 5
  constraint horizontal L23
  constraint vertical L24
  constraint horizontal L25
  constraint vertical L26
  constraint coincident L16.end L17.start
  constraint horizontal L27
  constraint vertical L28
  constraint horizontal L29
  constraint vertical L30
  constraint coincident L24 L31.end
  constraint perpendicular L24 L31
  constraint horizontal L32
  constraint vertical L33
  constraint horizontal L34
  constraint vertical L35
  constraint horizontal L36
  constraint vertical L37
  constraint horizontal L38
  constraint vertical L39
  measures "d181" distance of L16.end L17.end
  measures "d182" distance of L16.end L25.end
  measures "d185" distance of L24.end L27.end
  measures "d186" distance of L24.end L29.end
  measures "d188" distance of L31.start L31.end
  measures "d189" distance of L31.start L34.end
extrude "Extrude19" add sketch "Sketch20" along normal blind 18 contours A7 L24 L31 L32 L33 L35 L36 | L16 L17 L23 L24 L25 L26 L30 L33 L37 | L24 L29 L31 L32 L36 L37 L38 L39 | L24 L27 L28 L29 L30 L38 bodies 1
sketch "Sketch7" plane through (70, 0, 0) normal (1, 0, 0) x (0, 1, 0)
  line L0 (30, 0) -> (30, 20)
  line L1 (30, 20) -> (-30, 20)
  line L2 (-30, 20) -> (-30, 0)
  line L3 (-30, 0) -> (30, 0)
  line L4 (19.5, 20) -> (19.5, 0) construction
  line L5 (13.25, 9.25) -> (46, 9.25) construction
  line L6 (16.75, 7.25) -> (22.35, 7.25)
  arc A0 (22.35, 7.25) -> (22.35, 11.25) centre (22.35, 9.25) ccw
  line L7 (22.35, 11.25) -> (16.75, 11.25)
  arc A1 (16.75, 11.25) -> (16.75, 7.25) centre (16.75, 9.25) ccw
  line L8 (16.75, 9.25) -> (22.35, 9.25) construction
  line L9 (16.9, 5.6) -> (22.1, 5.6)
  arc A2 (22.1, 5.6) -> (22.1, 12.9) centre (22.1, 9.25) ccw
  line L10 (22.1, 12.9) -> (16.9, 12.9)
  arc A3 (16.9, 12.9) -> (16.9, 5.6) centre (16.9, 9.25) ccw
  line L11 (16.9, 9.25) -> (22.1, 9.25) construction
  point P0 (19.5, 9.25)
  point P1 (19.5, 9.25)
  dimension "d47" = 9.25
  dimension "d48" = 10.5
  dimension "d49" = 2.85
  dimension "d50" = 2
  dimension "d51" = 5.6
  dimension "d179" = 7.3
  dimension "d180" = 2.6
  constraint coincident L1 L4.start
  constraint perpendicular L1 L4
  constraint coincident L3 L4.end
  constraint perpendicular L4 L5
  constraint tangent L6 A0
  constraint tangent A0 L7
  constraint parallel L6 L7
  constraint tangent L7 A1
  constraint tangent L6 A1
  constraint perpendicular L4 L8
  constraint coincident L5 P1
  constraint coincident L4 P1
  constraint tangent L9 A2
  constraint tangent A2 L10
  constraint parallel L9 L10
  constraint tangent L10 A3
  constraint tangent L9 A3
  constraint coincident L5 A2.centre
  constraint perpendicular L4 L11
  constraint coincident P1 P0
  constraint midpoint L11 P1
  constraint coincident L8 A2.centre
  constraint midpoint L5.start A3
  measures "d47" distance of L3 L5
  measures "d48" distance of L0 L4
  measures "d49" distance of A0.centre P1
  measures "d50" distance of A0.end A0.centre
  measures "d51" distance of A1.centre A0.centre
  measures "d179" diameter of A2
  measures "d180" distance of P1 A2.centre
extrude "Extrude6" cut sketch "Sketch7" against normal blind 8 contours L6 A0 L7 A1 | L9 A2 L10 A3 bodies 1
sketch "Sketch21" plane through (0, 0, 2) normal (0, 0, 1) x (-1, 0, 0)
  circle A0 centre (-49.5, -19.5) radius 3
  circle A1 centre (21.9294, 25) radius 3
  circle A2 centre (5.9294, 25) radius 3
  line L0 (-68, -12) -> (-62, -12)
  line L1 (-62, -12) -> (-62, -33)
  line L2 (-62, -33) -> (62, -33)
  line L3 (62, -33) -> (62, -29)
  arc A3 (64, -27) -> (62, -29) centre (64, -29) ccw
  line L4 (64, -27) -> (68, -27)
  line L5 (68, -27) -> (68, 27)
  line L6 (68, 27) -> (53, 27)
  line L7 (53, 27) -> (53, 28)
  line L8 (53, 28) -> (62.2679, 28)
  arc A4 (62, 29) -> (62.2679, 28) centre (64, 29) ccw
  line L9 (62, 29) -> (62, 33)
  line L10 (62, 33) -> (-62, 33)
  line L11 (-62, 33) -> (-62, 2)
  line L12 (-68, 2) -> (-68, 1.5)
  line L13 (-68, 1.5) -> (-45, 1.5)
  line L14 (-45, 1.5) -> (-45, 0.5)
  line L15 (-45, 0.5) -> (-68, 0.5)
  line L16 (-68, 0.5) -> (-68, -12)
  circle A5 centre (5.9294, -25) radius 3
  circle A6 centre (21.9294, -25) radius 3
  circle A7 centre (13.9294, -15) radius 3
  circle A8 centre (13.9294, 15) radius 3
  line L17 (31.1094, 25.8906) -> (31.1094, 22.8906)
  line L18 (31.1094, 22.8906) -> (27.1094, 22.8906)
  line L19 (27.1094, 22.8906) -> (27.1094, 30.8906)
  line L20 (27.1094, 30.8906) -> (35.1094, 30.8906)
  line L21 (35.1094, 30.8906) -> (35.1094, 26.8906)
  line L22 (35.1094, 26.8906) -> (32.1094, 26.8906)
  arc A9 (32.1094, 26.8906) -> (31.1094, 25.8906) centre (32.1094, 25.8906) ccw
  circle A10 centre (-17.5, -19.5) radius 3
  circle A11 centre (58, -29) radius 2
  circle A12 centre (58, -29) radius 3
  line L23 (-62, 2) -> (-68, 2)
  dimension "d190" = 4
  dimension "d191" = 6
  dimension "d192" = 4
  dimension "d193" = 4
  constraint concentric A11 A12
  measures "d190" diameter of A11
  measures "d191" diameter of A12
  measures "d192" distance of L2 A11.centre
  measures "d193" distance of L3 A11.centre
extrude "Extrude20" add sketch "Sketch21" along normal blind 15.2 contours A12 bodies 1
sketch "Sketch24" plane through (0, 0, 2) normal (0, 0, 1) x (-1, 0, 0)
  circle A0 centre (-17.5, -19.5) radius 3
  line L0 (31.1094, 25.8906) -> (31.1094, 22.8906)
  line L1 (31.1094, 22.8906) -> (27.1094, 22.8906)
  line L2 (27.1094, 22.8906) -> (27.1094, 30.8906)
  line L3 (27.1094, 30.8906) -> (35.1094, 30.8906)
  line L4 (35.1094, 30.8906) -> (35.1094, 26.8906)
  line L5 (35.1094, 26.8906) -> (32.1094, 26.8906)
  arc A1 (32.1094, 26.8906) -> (31.1094, 25.8906) centre (32.1094, 25.8906) ccw
  circle A2 centre (13.9294, 15) radius 3
  circle A3 centre (13.9294, -15) radius 3
  circle A4 centre (21.9294, -25) radius 3
  circle A5 centre (5.9294, -25) radius 3
  line L6 (-68, -12) -> (-62, -12)
  line L7 (-62, -12) -> (-62, -33)
  line L8 (-62, -33) -> (62, -33)
  line L9 (62, -33) -> (62, -29)
  arc A6 (64, -27) -> (62, -29) centre (64, -29) ccw
  line L10 (64, -27) -> (68, -27)
  line L11 (68, -27) -> (68, 27)
  line L12 (68, 27) -> (53, 27)
  line L13 (53, 27) -> (53, 28)
  line L14 (53, 28) -> (62.2679, 28)
  arc A7 (62, 29) -> (62.2679, 28) centre (64, 29) ccw
  line L15 (62, 29) -> (62, 33)
  line L16 (62, 33) -> (-62, 33)
  line L17 (-62, 33) -> (-62, 2)
  line L18 (-62, 2) -> (-68, 2)
  line L19 (-68, 2) -> (-68, 1.5)
  line L20 (-68, 1.5) -> (-45, 1.5)
  line L21 (-45, 1.5) -> (-45, 0.5)
  line L22 (-45, 0.5) -> (-68, 0.5)
  line L23 (-68, 0.5) -> (-68, -12)
  circle A8 centre (5.9294, 25) radius 3
  circle A9 centre (21.9294, 25) radius 3
  circle A10 centre (-49.5, -19.5) radius 3
  circle A11 centre (58, -29) radius 3
  line L24 (0, 28) -> (-2, 28)
  line L25 (-2, 28) -> (-2, 6.5)
  line L26 (-2, 6.5) -> (0, 6.5)
  line L27 (0, 6.5) -> (0, 28)
  dimension "d205" = 21.5
  dimension "d206" = 5
  dimension "d207" = 2
  constraint horizontal L24
  constraint vertical L25
  constraint horizontal L26
  constraint vertical L27
  measures "d205" distance of L24.start L26.end
  measures "d206" distance of L16 L24
  measures "d207" distance of L24.start L24.end
extrude "Extrude23" add sketch "Sketch24" along normal blind 5 contours L24 L25 L26 L27 bodies 1
chamfer "Chamfer5" distance 2 angle 45 1 edges at (2, -17.25, 7) on bodies 1